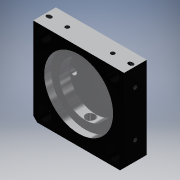
# Autodesk Inventor part: backlight (G061008000)
Saved by Autodesk Inventor 2017 (Build 210142000, 142)
## iProperties
Part Number: backlight (G061008000)
Material: Generisch
Document SubType Name: Modeling
Designer: David Merges
Density: 1 g/cm^3
Appearance: Eloxiert - schwarz
Author: David Merges
Autodesk Inventor part; units mm, degrees
note: some values were not read from the file. Chosen so that the rebuilt part matches the saved one: direction of "Bohrung4"; direction of "Bohrung8".
ref_plane "YZ Plane" through (0, 0, 0) normal (1, 0, 0) x (0, 1, 0)
ref_plane "XZ Plane" through (0, 0, 0) normal (0, 1, 0) x (-1, 0, 0)
ref_plane "XY Plane" through (0, 0, 0) normal (0, 0, 1) x (1, 0, 0)
sketch "Skizze1" plane through (0, 0, 0) normal (0, 1, 0) x (-1, 0, 0)
  line L0 (20, 20) -> (-20, 20)
  line L1 (-20, 20) -> (-20, -20)
  line L2 (-20, -20) -> (20, -20)
  line L3 (20, -20) -> (20, 20)
  line L4 (20, -20) -> (-20, 20) construction
  point P0 (0, 0)
  point P1 (0, 0)
  dimension "d0" = 40
  dimension "d1" = 40
  constraints: 10 end point, 2 parallel, 1 coincident, 1 horizontal, 1 midpoint, 1 perpendicular
  measures "d0" distance of L2.end L1.end
  measures "d1" distance of L1.end L0.end
extrude "Extrusion1" add sketch "Skizze1" along normal mid plane 10
sketch "Skizze2" plane through (0, -5, 0) normal (0, -1, 0) x (1, 0, 0)
  line L0 (-15, 15) -> (15, 15) construction
  line L1 (15, 15) -> (15, -15) construction
  line L2 (15, -15) -> (-15, -15) construction
  line L3 (-15, -15) -> (-15, 15) construction
  line L4 (15, -15) -> (-15, 15) construction
  point P0 (0, 0)
  dimension "d4" = 30
  dimension "d5" = 30
  constraints: 10 end point, 2 midpoint, 2 parallel, 1 horizontal, 1 perpendicular
  measures "d4" distance of L1.end L2.end
  measures "d5" distance of L0.end L1.end
hole "Bohrung1" at (15, -5, -15) at (15, -5, 15) at (-15, -5, 15) at (-15, -5, -15) direction (0, 1, 0) diameter 6 end through all
sketch "Skizze3" plane through (0, -5, 0) normal (0, -1, 0) x (1, 0, 0)
  circle A0 centre (-15, 15) radius 3 projected
  circle A1 centre (15, -15) radius 3 projected
  circle A2 centre (15, 15) radius 3 projected
  circle A3 centre (-15, -15) radius 3 projected
  line L0 (20, 20) -> (-20, 20) projected
  line L1 (-20, 20) -> (-20, -20) projected
  line L2 (-20, -20) -> (20, -20) projected
  line L3 (20, -20) -> (20, 20) projected
  line L4 (-20, 18.2322) -> (-18.2322, 20)
  line L5 (-20, 20) -> (20, 20) projected
  line L6 (20, 20) -> (-20, 20) projected
  line L7 (-18.2322, 20) -> (-20, 20)
  line L8 (-20, 20) -> (-20, 18.2322)
  point P0 (0, 0)
  dimension "d13" = 45
  dimension "d14" = 2.5
  constraints: 6 end point, 2 collinear, 2 point on line
  measures "d13" angle of L0 L4
  measures "d14" distance of L4.start L4.end
extrude "Extrusion2" cut sketch "Skizze3" against normal through all contours L4 L1 L0
pattern_circular "Runde Anordnung1" count 4 over 360 about axis through (0, -10, 0) along (0, 1, 0) of "Extrusion2"
sketch "Skizze8" plane through (0, -5, 0) normal (0, -1, 0) x (1, 0, 0)
  circle A0 centre (0, 0) radius 11.5
  dimension "d36" = 23
  constraints: 1 centre point, 1 coincident
  measures "d36" diameter of A0
extrude "Extrusion6" cut sketch "Skizze8" against normal blind 7.5
sketch "Skizze9" plane through (0, 2.5, 0) normal (0, -1, 0) x (1, 0, 0)
  line L0 (-9.77, 0) -> (9.77, 0) construction
  point P0 (0, 0)
  point P1 (0, 0)
  dimension "d46" = 19.54
  constraints: 3 coincident, 2 end point, 1 horizontal, 1 midpoint
  measures "d46" distance of L0.start L0.end
hole "Bohrung3" at (-9.77, 2.5, 0) at (9.77, 2.5, 0) direction (0, 1, 0) diameter 3 end through all
sketch "Skizze12" plane through (0, -5, 0) normal (0, -1, 0) x (1, 0, 0)
  circle A0 centre (0, 0) radius 15.15
  circle A1 centre (0, 0) radius 11.5 projected
  line L0 (-20, -18.2322) -> (-18.2322, -20) projected
  line L1 (-18.2322, -20) -> (18.2322, -20) projected
  line L2 (18.2322, -20) -> (20, -18.2322) projected
  line L3 (20, -18.2322) -> (20, 18.2322) projected
  line L4 (20, 18.2322) -> (18.2322, 20) projected
  line L5 (18.2322, 20) -> (-18.2322, 20) projected
  line L6 (-18.2322, 20) -> (-20, 18.2322) projected
  line L7 (-20, 18.2322) -> (-20, -18.2322) projected
  circle A2 centre (-15, 15) radius 3 projected
  circle A3 centre (15, -15) radius 3 projected
  circle A4 centre (15, 15) radius 3 projected
  circle A5 centre (-15, -15) radius 3 projected
  dimension "d57" = 23
  dimension "d58" = 30.3
  constraints: 1 centre point, 1 coincident
  measures "d57" diameter of A1
  measures "d58" diameter of A0
extrude "Extrusion8" cut sketch "Skizze12" against normal blind 3 contours A0
sketch "Skizze10" plane through (18.2322, 5, -20) normal (0, 0, -1) x (-1, 0, 0)
  line L0 (36.4645, -10) -> (36.4645, 0) projected
  line L1 (0, 0) -> (36.4645, 0) projected
  line L2 (0, 0) -> (0, -10) projected
  line L3 (36.4645, -10) -> (0, -10) projected
  line L4 (29.7322, -2.5) -> (6.7322, -2.5) projected
  line L5 (29.7322, -10) -> (6.7322, -10) projected
  line L6 (6.7322, -7) -> (29.7322, -7) projected
  line L7 (33.3822, -7) -> (3.0822, -7) projected
  line L8 (29.5022, -2.5) -> (26.5022, -2.5) projected
  line L9 (9.9622, -2.5) -> (6.9622, -2.5) projected
  line L10 (29.7322, -2.5) -> (6.7322, -2.5) projected
  line L11 (18.2322, -7) -> (18.2322, -2.5)
  point P0 (18.2322, -5)
  point P1 (18.2322, -4.75)
  point P2 (18.2322, -4.75)
  point P3 (18.2322, -4.75)
  constraints: 3 midpoint, 2 coincident, 2 end point, 1 perpendicular, 2 other
hole "Bohrung4" at (0, 0.25, -20) direction (0, 0, 1) diameter 4.2 end up to surface
sketch "Skizze15" plane through (-18.2322, -5, 20) normal (0, 0, 1) x (1, 0, 0)
  line L0 (38.2322, 10) -> (38.2322, 0) projected
  line L1 (-1.7678, 0) -> (-1.7678, 10) projected
  line L2 (-1.7678, 10) -> (-1.7678, 0) construction
  line L3 (38.2322, 10) -> (36.4645, 10) construction
  line L4 (-1.7678, 0) -> (38.2322, 10) construction
  line L5 (8.2322, 5) -> (28.2322, 5) construction
  point P0 (18.2322, 5)
  point P1 (18.2322, 5)
  dimension "d85" = 20
  constraints: 4 end point, 2 coincident, 2 midpoint, 1 perpendicular
  measures "d85" distance of L5.start L5.end
hole "Bohrung7" at (-10, 0, 20) at (10, 0, 20) direction (0, 0, -1) diameter 1.813 depth 10 tip angle 118 thread size "M2.3x0.45" class "6H" standard "ISO Metric profile"
pattern_circular "Runde Anordnung2" count 4 over 360 about axis through (0, -10, 0) along (0, 1, 0) of "Bohrung7"
sketch "Skizze16" plane through (18.2322, -5, 20) normal (0.7071068, 0, 0.7071068) x (0.7071068, 0, -0.7071068)
  line L0 (2.5, 0) -> (0, 0) projected
  line L1 (0, 10) -> (2.5, 10) projected
  line L2 (0, 10) -> (0, 0) construction
  line L3 (2.5, 0) -> (2.5, 10) construction
  line L4 (0, 0) -> (2.5, 10) construction
  point P0 (1.25, 5)
  point P1 (1.25, 5)
  constraints: 2 end point, 1 coincident
hole "Bohrung8" at (19.1161, 0, 19.1161) direction (-0.7071068, 0, -0.7071068) diameter 1.813 end up to surface thread size "M2.3x0.45" class "6H" standard "ISO Metric profile"
pattern_circular "Runde Anordnung3" count 4 over 360 about axis through (0, -10, 0) along (0, 1, 0) of "Bohrung8"
sketch "Skizze17" plane through (18.2322, 5, -20) normal (0, 0, -1) x (-1, 0, 0)
  circle A0 centre (28.2322, -5) radius 0.9065 projected
  circle A1 centre (8.2322, -5) radius 0.9065 projected
  circle A2 centre (18.2322, -4.75) radius 2.1 projected
  line L0 (36.4645, -10) -> (36.4645, 0) projected
  line L1 (0, 0) -> (36.4645, 0) projected
  line L2 (0, 0) -> (0, -10) projected
  line L3 (36.4645, -10) -> (0, -10) projected
  circle A3 centre (9.8257, -5) radius 2.5
  line L4 (8.2322, -5) -> (9.8257, -5)
  line L5 (36.4645, -10) -> (0, -10) projected
  circle A4 centre (8.2322, -5) radius 0.9065 projected
  point P0 (18.2322, -5)
  dimension "d107" = 5
  constraints: 2 end point, 1 centre point, 1 parallel, 1 tangent
  measures "d107" diameter of A3
extrude "Extrusion9" cut sketch "Skizze17" against normal blind 5 contours A3
sketch "Skizze18" plane through (-18.2322, -5, 20) normal (0, 0, 1) x (1, 0, 0)
  line L0 (-16.0679, -9.1874) -> (50.249, -9.1874)
  line L1 (50.249, -9.1874) -> (50.249, 27.2367)
  line L2 (50.249, 27.2367) -> (-16.0679, 27.2367)
  line L3 (-16.0679, 27.2367) -> (-16.0679, -9.1874)
  point P0 (18.2322, 5)
  constraints: 8 end point, 2 parallel, 1 horizontal, 1 perpendicular
extrude "Extrusion10" cut sketch "Skizze18" against normal blind 2
